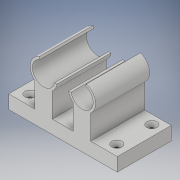
# Autodesk Inventor part: Part1
Saved by Autodesk Inventor 2018 (Build 220112000, 112)
## iProperties
Created: 2019-04-30
Part Number: Part1
Material: Generic
Document SubType Name: Modeling
Designer: F8PLTW
Density: 1 g/cm^3
Appearance: Default
Author: F8PLTW
Autodesk Inventor part; units mm, degrees
ref_plane "YZ Plane" through (0, 0, 0) normal (1, 0, 0) x (0, 1, 0)
ref_plane "XZ Plane" through (0, 0, 0) normal (0, 1, 0) x (-1, 0, 0)
ref_plane "XY Plane" through (0, 0, 0) normal (0, 0, 1) x (1, 0, 0)
sketch "Sketch1" plane through (0, 0, 0) normal (0, 0, 1) x (1, 0, 0)
  arc A0 (-13.2818, 11.9603) -> (-0.6453, -3.2505) centre (-9.7741, 2.02) ccw
  line L0 (-9.7741, 2.02) -> (-0.6453, 7.2905) construction
  line L1 (-9.7741, 2.02) -> (0.7669, 2.02) construction
  line L2 (-9.7741, 2.02) -> (-0.6453, -3.2505) construction
  line L3 (-9.7741, 2.02) -> (0.7669, 2.02) construction
  line L4 (8.2613, 16.5876) -> (8.2613, -12.065) construction
  line L5 (-13.2818, 11.9603) -> (-14.0002, 13.9962)
  arc A1 (-13.2818, 11.9603) -> (0.5715, 0) centre (-9.7741, 2.02) ccw
  line L6 (0.5715, 0) -> (2.7642, 0)
  arc A2 (17.168, -3.2505) -> (29.8044, 11.9603) centre (26.2967, 2.02) ccw
  line L7 (29.8044, 11.9603) -> (30.5229, 13.9962)
  arc A3 (15.9511, 0) -> (29.8044, 11.9603) centre (26.2967, 2.02) ccw
  line L8 (15.9511, 0) -> (13.7584, 0)
  line L9 (-17.9133, -7.729) -> (-17.9133, -30.6279)
  line L10 (-17.9133, -30.6279) -> (-1.615, -30.6279)
  line L11 (-1.615, -30.6279) -> (-1.615, -7.7124)
  line L12 (34.436, -7.729) -> (34.436, -30.6279)
  line L13 (34.436, -30.6279) -> (18.1376, -30.6279)
  line L14 (18.1376, -30.6279) -> (18.1376, -7.7124)
  arc A4 (13.7584, 0) -> (18.1376, -7.7124) centre (26.2967, 2.02) ccw
  arc A5 (34.436, -7.729) -> (30.5229, 13.9962) centre (26.2967, 2.02) ccw
  arc A6 (15.2982, -4.33) -> (18.1376, -7.7124) centre (26.2967, 2.02) ccw
  arc A7 (34.436, -7.729) -> (30.5229, 13.9962) centre (26.2967, 2.02) ccw
  arc A8 (-14.0002, 13.9962) -> (-17.9133, -7.729) centre (-9.7741, 2.02) ccw
  arc A9 (-1.615, -7.7124) -> (1.2244, -4.33) centre (-9.7741, 2.02) ccw
  arc A10 (-14.0002, 13.9962) -> (-17.9133, -7.729) centre (-9.7741, 2.02) ccw
  arc A11 (-1.615, -7.7124) -> (2.7642, 0) centre (-9.7741, 2.02) ccw
  point P0 (0, 0)
  dimension "d0" = 21.082
  dimension "d2" = 30
  dimension "d3" = 30
  constraints: 30 end point, 28 point on circle, 14 symmetric about line, 12 centre point, 6 coincident, 3 horizontal, 2 equal length, 2 perpendicular, 2 vertical, 2 other
  measures "d0" diameter of A0
  measures "d2" angle of L1 L0
  measures "d3" angle of L2 L3
extrude "Extrusion1" add sketch "Sketch1" along normal blind 50.8
sketch "Sketch2" plane through (-17.9133, -30.6279, 0) normal (0, -1, 0) x (1, 0, 0)
  line L0 (-24.7177, 50.8) -> (77.3849, 50.8)
  line L1 (77.3849, 50.8) -> (77.3849, 0)
  line L2 (77.3849, 0) -> (-24.7177, 0)
  line L3 (-24.7177, 0) -> (-24.7177, 50.8)
  point P0 (17.9133, 0)
  constraints: 8 end point, 2 parallel, 1 horizontal, 1 perpendicular
extrude "Extrusion2" add sketch "Sketch2" along normal blind 12.7
sketch "Sketch3" plane through (-17.9133, -30.6279, 0) normal (0, 1, 0) x (1, 0, 0)
  point P0 (17.9133, 0)
sketch "Sketch4" plane through (-17.9133, -30.6279, 0) normal (0, 1, 0) x (1, 0, 0)
  point P0 (17.9133, 0)
hole "Hole1" at (49.2151, -30.6279, 40.9398) direction (0, -1, 0) diameter 3.556 end through all countersink diameter 9.525 countersink angle 82
hole "Hole2" at (49.7086, -30.6279, 8.5342) direction (0, -1, 0) diameter 3.556 end through all countersink diameter 9.525 countersink angle 82
hole "Hole3" at (-32.3747, -30.6279, 40.9398) direction (0, -1, 0) diameter 3.556 end through all countersink diameter 9.525 countersink angle 82
hole "Hole4" at (-32.2102, -30.6279, 8.5342) direction (0, -1, 0) diameter 3.556 end through all countersink diameter 9.525 countersink angle 82
thread "Thread1" size "6-32 UNC" class "2B" standard "ANSI Unified Screw Threads" full length
thread "Thread2" size "6-32 UNC" class "2B" standard "ANSI Unified Screw Threads" full length
thread "Thread3" size "8-32 UNC" class "2B" standard "ANSI Unified Screw Threads" full length
thread "Thread4" size "6-32 UNC" class "2B" standard "ANSI Unified Screw Threads" full length
thread "Thread5" size "6-32 UNC" class "2B" standard "ANSI Unified Screw Threads" full length
thread "Thread6" size "6-32 UNC" class "2B" standard "ANSI Unified Screw Threads" full length
body "Solid1"
